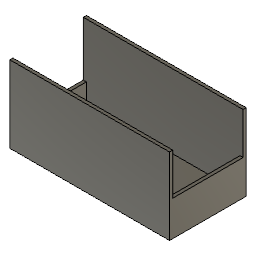
imaging_stand_light_shield (Autodesk Fusion 360 design; units mm, degrees)
Autodesk Fusion 360 part; units mm, degrees
sketch "スケッチ1" plane through (0, 0, 0) normal (0, 0, 1) x (1, 0, 0)
  line L0 (125, -60) -> (-125, -60)
  line L1 (-125, -60) -> (-125, 60)
  line L2 (-125, 60) -> (125, 60)
  line L3 (125, 60) -> (125, -60)
  line L4 (125, -60) -> (-125, 60) construction
  line L5 (-125, -60) -> (125, 60) construction
  dimension "d1" = 250
  dimension "d2" = 120
  constraint horizontal L0
  constraint perpendicular L0 L1
  constraint parallel L0 L2
  constraint parallel L1 L3
  constraint coincident L4 origin
  constraint coincident L5 origin
  measures "d1" distance of L1.end L2.end
  measures "d2" distance of L0.end L1.end
extrude "押し出し1" add sketch "スケッチ1" along normal blind 120
sketch "スケッチ2" plane through (0, 0, 120) normal (0, 0, 1) x (-1, 0, 0)
  line L0 (-125, -60) -> (125, -60)
  line L1 (125, -60) -> (125, 60)
  line L2 (125, 60) -> (-125, 60)
  line L3 (-125, 60) -> (-125, -60)
  line L4 (-125, 55) -> (125, 55)
  line L5 (125, 55) -> (125, -55)
  line L6 (125, -55) -> (-125, -55)
  line L7 (-125, -55) -> (-125, 55)
  line L8 (-125, 55) -> (125, -55) construction
  line L9 (125, 55) -> (-125, -55) construction
  dimension "d5" = 250
  dimension "d6" = 110
  constraint horizontal L4
  constraint perpendicular L4 L5
  constraint parallel L4 L6
  constraint parallel L5 L7
  constraint coincident L8 origin
  constraint coincident L9 origin
  measures "d5" distance of L5.end L6.end
  measures "d6" distance of L4.end L5.end
extrude "押し出し2" cut sketch "スケッチ2" against normal blind 115 contours L1 L3 L4 L5 L6 L7
sketch "スケッチ3" plane through (0, 0, 5) normal (0, 0, 1) x (-1, 0, 0)
  line L0 (-125, -55) -> (125, -55)
  line L1 (125, -55) -> (125, 55)
  line L2 (125, 55) -> (-125, 55)
  line L3 (-125, 55) -> (-125, -55)
  line L4 (-125, -55) -> (-120, -55)
  line L5 (-120, -55) -> (-120, 55)
  line L6 (-120, 55) -> (-125, 55)
  line L7 (-125, 55) -> (-125, -55)
  constraint horizontal L4
  constraint vertical L5
  constraint horizontal L6
  constraint vertical L7
  constraint coincident L0.start L3.end
extrude "押し出し3" add sketch "スケッチ3" along normal blind 50 contours L0 L2 L3 L4 L5 L6 L7
sketch "スケッチ4" plane through (0, 0, 5) normal (0, 0, 1) x (-1, 0, 0)
  line L0 (-120, 55) -> (-120, -55)
  line L1 (-120, -55) -> (125, -55)
  line L2 (125, -55) -> (125, 55)
  line L3 (125, 55) -> (-120, 55)
  line L4 (120, -55) -> (125, -55)
  line L5 (125, -55) -> (125, 55)
  line L6 (125, 55) -> (120, 55)
  line L7 (120, 55) -> (120, -55)
  constraint horizontal L4
  constraint vertical L5
  constraint horizontal L6
  constraint vertical L7
  constraint coincident L2.end L3.start
  constraint coincident L1 L4.start
extrude "押し出し4" add sketch "スケッチ4" along normal blind 30 contours L1 L2 L3 L4 L5 L6 L7
